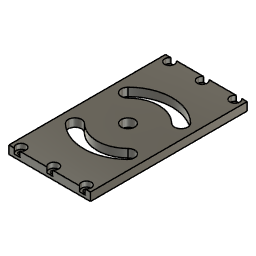
FS80 Pivot Base v5 (Autodesk Fusion 360 design; units mm, degrees)
Autodesk Fusion 360 part; units mm, degrees
sketch "Schizzo5" plane through (0, 0, 0) normal (0, 0, 1) x (1, 0, 0)
  line L0 (84.2066, 82.4519) -> (84.2066, -13.5481)
  circle A0 centre (89.2066, -11.0481) radius 1.5
  circle A1 centre (129.2066, 79.9519) radius 3
  line L1 (84.2066, 34.4519) -> (134.2066, 34.4519) construction
  circle A2 centre (109.2066, 79.9519) radius 1.5
  circle A3 centre (89.2066, 79.9519) radius 3
  circle A4 centre (89.2066, 79.9519) radius 1.5
  line L2 (134.2066, 82.4519) -> (84.2066, 82.4519)
  circle A5 centre (129.2066, 79.9519) radius 1.5
  circle A6 centre (109.2066, 79.9519) radius 3
  circle A7 centre (109.2066, 34.4519) radius 4.1
  circle A8 centre (109.2066, -11.0481) radius 1.5
  line L3 (134.2066, -13.5481) -> (134.2066, 82.4519)
  line L4 (89.2066, 82.4519) -> (89.2066, -13.5481) construction
  circle A9 centre (89.2066, -11.0481) radius 3
  circle A10 centre (109.2066, -11.0481) radius 3
  circle A11 centre (129.2066, -11.0481) radius 1.5
  line L5 (84.2066, -13.5481) -> (134.2066, -13.5481)
  circle A12 centre (129.2066, -11.0481) radius 3
  line L6 (84.2066, -11.0481) -> (134.2066, -11.0481) construction
  line L7 (109.2066, 82.4519) -> (109.2066, -13.5481) construction
  line L8 (109.2066, 34.4519) -> (109.2066, 59.4519) construction
  line L9 (109.2066, 34.4519) -> (109.2066, 59.4519) construction
  line L10 (109.2066, 34.4519) -> (92.9431, 18.1884) construction
  circle A13 centre (92.9431, 18.1884) radius 4.1
  circle A14 centre (92.9431, 50.7153) radius 4.1
  circle A15 centre (125.47, 50.7153) radius 4.1
  circle A16 centre (125.47, 18.1884) radius 4.1
  circle A17 centre (109.2066, 34.4519) radius 18.9
  circle A18 centre (109.2066, 34.4519) radius 27.1
  point P0 (127.8474, 12.2366)
  dimension "d221" = 50
  dimension "d222" = 96
  dimension "d223" = 2.5
  dimension "d224" = 20
  dimension "d225" = 3
  dimension "d226" = 6
  dimension "d227" = 3
  dimension "d228" = 6
  dimension "d229" = 8.2
  dimension "d350" = 8.2
  dimension "d351" = 45
  dimension "d352" = 23
  constraint horizontal L5
  constraint vertical L3
  constraint horizontal L2
  constraint vertical L0
  constraint midpoint L7.start L2
  constraint midpoint L7.end L5
  constraint coincident L6.end L3
  constraint perpendicular L3 L6
  constraint midpoint L1.start L0
  constraint midpoint L1.end L3
  constraint coincident L4.start L2
  constraint coincident L4.end L5
  constraint perpendicular L4 L5
  constraint coincident A0.centre L6
  constraint coincident A0.centre L4
  constraint concentric A0 A9
  constraint symmetric A0 A11 L7
  constraint symmetric A9 A12 L7
  constraint symmetric A0 L1 A4
  constraint symmetric L1 A3 A9
  constraint symmetric L1 A5 A11
  constraint symmetric A1 L1 A12
  constraint coincident A8.centre L7
  constraint coincident A8.centre L6
  constraint concentric A8 A10
  constraint symmetric L1 A2 A8
  constraint symmetric L1 A6 A10
  constraint midpoint A7.centre L1
  constraint coincident L8.end L7
  constraint coincident A7.centre L8.start
  constraint coincident L6.start L0
  constraint coincident L10.end A13.centre
  constraint symmetric L1 A13 A14
  constraint symmetric L7 A13 A16
  constraint symmetric L7 A14 A15
  constraint tangent A16 A17
  constraint concentric A17 A18
  constraint tangent A16 A18
  measures "d221" distance of L0.end L3.start
  measures "d222" distance of L0.end L0.start
  measures "d223" distance of L5 L6
  measures "d224" distance of L4 L7
  measures "d225" diameter of A0
  measures "d226" diameter of A9
  measures "d227" diameter of A8
  measures "d228" diameter of A10
  measures "d229" diameter of A7
  measures "d350" diameter of A13
  measures "d351" angle of L7 L10
  measures "d352" distance of A7.centre L10.end
extrude "Estrusione24" add sketch "Schizzo5" along normal blind 5 contours L0 A1 A3 L2 A6 L3 A18 | L0 A13 A14 A17 A18 | L0 L3 A9 A10 L5 A12 A18 | A17 | L3 A15 A16 A17 A18
extrude "Estrusione25" add sketch "Schizzo5" along normal blind 1.8 contours A3 L2 | L2 A6 | A9 L5 | A1 L2 | A10 L5 | L5 A12 picked at (89.244, 82.1172) picked at (109.244, 82.1172) picked at (89.244, -13.2134) picked at (129.244, 82.1172) picked at (109.244, -13.2134) picked at (129.244, -13.2134)
equation "d225 = d227"
equation "d226 = d228"
equation "d350 = d229"
named bodies: "Base"
